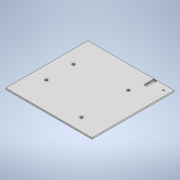
# Autodesk Inventor part: FitmentCard
Saved by Autodesk Inventor 2020.3 (Build 243373000, 373)
## iProperties
Created: 2021-01-23
Part Number: FitmentCard
Material: Generic
Document SubType Name: Modeling
Designer: allofus
Density: 1 g/cm^3
Appearance: Default
Author: allofus
Autodesk Inventor part; units mm, degrees
ref_plane "YZ Plane" through (0, 0, 0) normal (1, 0, 0) x (0, 1, 0)
ref_plane "XZ Plane" through (0, 0, 0) normal (0, 1, 0) x (-1, 0, 0)
ref_plane "XY Plane" through (0, 0, 0) normal (0, 0, 1) x (1, 0, 0)
sketch "Sketch1" plane through (0, 0, 0) normal (0, 1, 0) x (-1, 0, 0)
  line L0 (0, 0) -> (0, 53.3)
  line L1 (0, 53.3) -> (68.5346, 53.3)
  line L2 (68.5346, 53.3) -> (68.5346, 0)
  line L3 (68.5346, 0) -> (0, 0)
  line L4 (68.5346, 0) -> (68.5346, 2.5)
  line L5 (68.5346, 2.5) -> (68.5346, 7.6)
  line L6 (68.5346, 7.6) -> (68.5346, 35.5)
  line L7 (0, 53.3) -> (14, 53.3)
  line L8 (68.5346, 35.5) -> (68.5346, 50.7)
  circle A0 centre (13.5, 50.7) radius 1.4
  circle A1 centre (13.5, 2.5) radius 1.4
  circle A2 centre (64.8, 35.5) radius 1.4
  circle A3 centre (64.8, 7.6) radius 1.4
  line L9 (0, 63.3) -> (78.5346, 63.3)
  line L10 (78.5346, 63.3) -> (78.5346, 0)
  line L11 (-10, 53.3) -> (-10, -10)
  line L12 (-10, -10) -> (68.5346, -10)
  line L13 (-10, -10) -> (78.5346, -10)
  line L14 (78.5346, -10) -> (78.5346, 63.3)
  line L15 (78.5346, 63.3) -> (-10, 63.3)
  line L16 (-10, 63.3) -> (-10, -10)
  line L17 (74.5346, 63.3) -> (74.5346, -6)
  line L18 (74.5346, -6) -> (-10, -6)
  line L19 (78.5346, 59.3) -> (-6, 59.3)
  line L20 (-6, 59.3) -> (-6, -10)
  line L21 (14.5, 50.7) -> (14.5, 2.5)
  dimension "d0" = 53.3
  dimension "d1" = 68.5346
  dimension "d2" = 2.8
  dimension "d3" = 2.8
  dimension "d4" = 2.8
  dimension "d5" = 2.8
  dimension "d6" = 10
  dimension "d7" = 10
  dimension "d8" = 4
  dimension "d9" = 4
  dimension "d10" = 1
  dimension "d11" = 1
  constraints: 44 end point, 5 perpendicular, 5 point on line, 4 centre point, 2 horizontal, 2 parallel, 2 vertical, 4 other
  measures "d0" distance of L3.end L1.start
  measures "d1" distance of L1.start L1.end
  measures "d2" diameter of A0
  measures "d3" diameter of A1
  measures "d4" diameter of A2
  measures "d5" diameter of A3
  measures "d6" distance between parallel lines of L1 L9
  measures "d7" distance between parallel lines of L0 L11
  measures "d8" distance between parallel lines of L14 L17
  measures "d9" distance between parallel lines of L15 L19
  measures "d10" distance of A0.centre L21.start
  measures "d11" distance of A1.centre L21.end
extrude "Extrusion1" add sketch "Sketch1" along normal blind 1.5 contours L0 L1 L2 L3 | L9 L17 L19 L20 L18 L11 L16 L15 | L9 L10 L19 L17 | L19 L10 L14 L13 L12 L20 L18 L17 | L17 L18 L20 L19 | L18 L20 L12 L11
sketch "Sketch3" plane through (0, 1.5, 0) normal (0, 1, 0) x (1, 0, 0)
  line L0 (10, -63.3) -> (10, 10) projected
  line L1 (10, 10) -> (-78.5346, 10)
  line L2 (-78.5346, 10) -> (-78.5346, 21)
  line L3 (-78.5346, 21) -> (10, 21)
  line L4 (10, 21) -> (10, 10)
  line L5 (10, 21) -> (4.5, 21)
  line L6 (4.5, 21) -> (4.5, 15.5)
  line L7 (4.5, 15.5) -> (10, 15.5)
  line L8 (10, 15.5) -> (10, 21)
  circle A0 centre (4.5, 15.5) radius 0.8
  point P0 (0, 0)
  dimension "d14" = 11
  dimension "d15" = 5.5
  dimension "d16" = 5.5
  dimension "d17" = 1.6
  constraints: 16 end point, 4 parallel, 2 horizontal, 2 perpendicular, 1 centre point, 1 coincident
  measures "d14" distance of L1.end L2.end
  measures "d15" distance of L7.end L6.end
  measures "d16" distance of L6.end L5.end
  measures "d17" diameter of A0
extrude "Extrusion2" add sketch "Sketch3" against normal blind 1.5 contours L1 L2 L3 L6 A0 L7 L4 | L7 A0 L6 L3 L4
sketch "Sketch4" plane through (0, 1.5, 0) normal (0, 1, 0) x (1, 0, 0)
  circle A0 centre (4.5, 15.5) radius 0.8 projected
  line L0 (8.7, 15.5) -> (8.7, 20.5)
  line L1 (8.7, 20.5) -> (-11.3, 20.5)
  line L2 (-11.3, 20.5) -> (-11.3, 10.5)
  line L3 (-11.3, 10.5) -> (8.7, 10.5)
  line L4 (8.7, 10.5) -> (8.7, 15.5)
  line L5 (-11.3, 10.5) -> (-11.3, 20.5)
  line L6 (-10.3, 20.5) -> (-10.3, 10.5)
  line L7 (-6.3, 20.5) -> (-6.3, 10.5)
  line L8 (-7.3, 20.5) -> (-7.3, 10.5)
  point P0 (0, 0)
  dimension "d21" = 5
  dimension "d22" = 20
  dimension "d23" = 10
  dimension "d24" = 1
  dimension "d25" = 4
  dimension "d26" = 1
  constraints: 18 end point, 4 equal length, 4 perpendicular, 1 point on line
  measures "d21" distance of L0.start L0.end
  measures "d22" distance of L0.end L1.end
  measures "d23" distance of L1.end L2.end
  measures "d24" distance between parallel lines of L2 L6
  measures "d25" distance between parallel lines of L6 L7
  measures "d26" distance between parallel lines of L7 L8
extrude "Extrusion3" cut sketch "Sketch4" against normal blind 15.4 contours L8 L3 L6 L1
body "Solid1"
